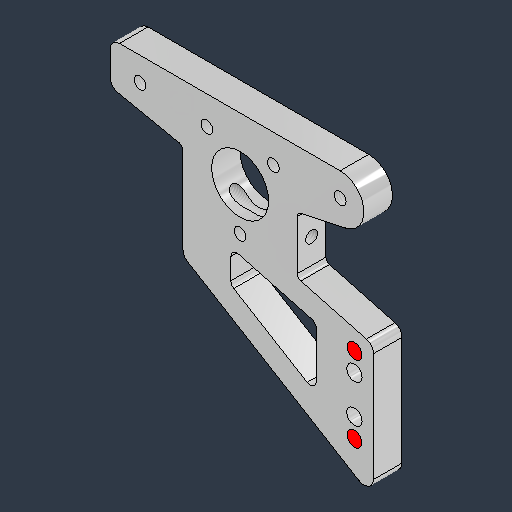
# Autodesk Inventor part: PLATE,SIDE,ELEVATOR,STAGE1
Saved by Autodesk Inventor 2024.3 (Build 283343000, 343)
## iProperties
ILogicPurgeVersion: 0.0.0.0
OnSaveVersion: 3.4.3.0
OnSaveAssembly: COREAutomationManager
Created: 2025-01-27
Part Number: PLATE,SIDE,ELEVATOR,STAGE1
Material: Aluminum 7075
Document SubType Name: Modeling
Designer: Jthib
Density: 2.81 g/cm^3
Appearance: Aluminum - Polished
Mfg Approved By: John.Thibert
Sheet Metal Rule: Default
Mass: 86.4188 g
Surface Area: 127.948 cm^2
Volume: 30.754 cm^3
ModelCat: Uncategorized
MaterialName: Aluminum 7075
CN_MASS: 0.09
Author: Jthib
Autodesk Inventor part; units mm, degrees
ref_plane "YZ Plane" through (0, 0, 0) normal (1, 0, 0) x (0, 1, 0)
ref_plane "XZ Plane" through (0, 0, 0) normal (0, 1, 0) x (-1, 0, 0)
ref_plane "XY Plane" through (0, 0, 0) normal (0, 0, 1) x (1, 0, 0)
sketch "Sketch1" plane through (0, 0, 0) normal (0, 0, 1) x (1, 0, 0)
  line L0 (33.401, 0) -> (-33.401, 0) construction
  arc A0 (33.401, 7.9375) -> (35.033, -7.7679) centre (33.401, 0) ccw construction
  arc A1 (-35.033, -7.7679) -> (-33.401, 7.9375) centre (-33.401, 0) ccw construction
  line L1 (33.401, 7.9375) -> (-33.401, 7.9375)
  line L2 (35.033, -7.7679) -> (19.1135, -11.1125)
  line L3 (19.1135, -11.1125) -> (19.1135, -30.1625)
  line L4 (19.1135, -30.1625) -> (44.5135, -36.9684)
  line L5 (44.5135, -36.9684) -> (44.5135, -81.4184)
  line L6 (44.5135, -81.4184) -> (-19.1135, -42.8625)
  line L7 (-19.1135, -42.8625) -> (-19.1135, -11.1125)
  line L8 (-19.1135, -11.1125) -> (-43.434, -6.0029)
  arc A2 (35.033, -7.7679) -> (33.401, 7.9375) centre (33.401, 0) ccw
  arc A3 (-33.401, 7.9375) -> (-35.033, -7.7679) centre (-33.401, 0) ccw
  line L9 (0, 26.6914) -> (0, -99.4367) construction
  line L10 (-33.401, 7.9375) -> (-43.434, 7.9375)
  line L11 (-43.434, 7.9375) -> (-43.434, -6.0029)
  point P0 (0, 0)
  point P1 (0, 0)
  point P2 (19.1135, -20.6375)
  dimension "d24" = 50.927
  dimension "d25" = 7.9375
  dimension "d26" = 19.05
  dimension "d27" = 19.05
  dimension "d28" = 105
  dimension "d30" = 6.35
  dimension "d31" = 44.45
  dimension "d72" = 28.575
  dimension "d110" = 31.75
  dimension "d127" = 10.033
  constraints: 22 end point, 8 point on circle, 6 tangent, 5 coincident, 4 centre point, 2 horizontal, 2 midpoint, 2 parallel, 1 equal radius, 1 perpendicular, 1 point on line, 1 vertical, 2 other
  measures "d25" radius of A2
  measures "d26" distance of L2.end L3.end
  measures "d28" angle of L3 L4
  measures "d30" distance edge to line of A0 L3
  measures "d31" distance of L4.end L5.end
  measures "d72" distance from line of L1 point (19.114, -20.638)
  measures "d110" distance of L6.end L7.end
  measures "d127" distance from line of L11 L0.end
extrude "Extrusion2" add sketch "Sketch1" along normal mid plane 9.525
sketch "Sketch2" plane through (0, 0, 4.7625) normal (0, 0, 1) x (1, 0, 0)
  arc A0 (35.033, -7.7679) -> (33.401, 7.9375) centre (33.401, 0) ccw construction
  line L0 (33.401, 0) -> (-33.401, 0) construction
  point P0 (0, 0)
  point P1 (0, 0)
  constraints: 3 coincident, 2 end point, 1 horizontal, 1 midpoint
hole "Hole1" at (33.401, 0, 4.7625) at (-33.401, 0, 4.7625) direction (0, 0, -1) diameter 3.9624 end through all thread size "10-32 UNF" class "2B" standard "ANSI Unified Screw Threads"
sketch "Sketch3" plane through (0, 0, -4.7625) normal (0, 0, -1) x (-1, 0, 0)
  line L0 (-62.103, 0) -> (61.0235, 0) construction
  line L1 (0, -99.2896) -> (0, 25.8087) construction
  line L2 (11.1125, -1.5875) -> (-11.1125, -1.5875) construction
  line L3 (0, -26.9875) -> (0, -1.5875) construction
  point P0 (0, 0)
  dimension "d43" = 22.225
  dimension "d44" = 25.4
  dimension "d45" = 1.5875
  constraints: 4 end point, 3 coincident, 1 collinear, 1 horizontal, 1 midpoint
  measures "d43" distance of L2.start L2.end
  measures "d44" distance of L3.start L3.end
  measures "d45" distance between parallel lines of L0 L2
hole "Hole2" at (0, -26.9875, -4.7625) at (11.1125, -1.5875, -4.7625) at (-11.1125, -1.5875, -4.7625) direction (0, 0, 1) diameter 3.9624 end through all thread size "10-32 UNF" class "2B" standard "ANSI Unified Screw Threads"
sketch "Sketch4" plane through (0, 0, 4.7625) normal (0, 0, 1) x (1, 0, 0)
  line L0 (0, 0) -> (0, -12.7) construction
  circle A0 centre (0, -12.7) radius 9.525
  line L1 (25.4635, -56.9863) -> (25.4635, -41.6407)
  line L2 (23.9574, -39.6779) -> (-0.5536, -33.1102)
  line L3 (-3.1115, -35.073) -> (-3.1115, -42.1335)
  line L4 (-2.1326, -43.8713) -> (22.3784, -58.7242)
  line L5 (-19.1135, -42.8625) -> (44.5135, -81.4184) construction
  line L6 (44.5135, -36.9684) -> (19.1135, -30.1625) construction
  line L7 (44.5135, -81.4184) -> (44.5135, -36.9684) construction
  arc A1 (22.3784, -58.7242) -> (25.4635, -56.9863) centre (23.4315, -56.9863) ccw
  arc A2 (25.4635, -41.6407) -> (23.9574, -39.6779) centre (23.4315, -41.6407) ccw
  arc A3 (-0.5536, -33.1102) -> (-3.1115, -35.073) centre (-1.0795, -35.073) ccw
  arc A4 (-3.1115, -42.1335) -> (-2.1326, -43.8713) centre (-1.0795, -42.1335) ccw
  point P0 (-18.2864, -30.0929)
  point P1 (20.2266, -29.9445)
  point P2 (19.1135, -30.1625)
  dimension "d54" = 19.05
  dimension "d55" = 12.7
  dimension "d56" = 19.05
  dimension "d57" = 28.575
  dimension "d58" = 7.9375
  dimension "d59" = 7.9375
  dimension "d60" = 2.032
  constraints: 10 end point, 8 point on circle, 8 tangent, 5 centre point, 3 equal radius, 2 vertical, 1 coincident, 1 parallel, 4 other
  measures "d54" diameter of A0
  measures "d55" distance of L0.start L0.end
  measures "d56" distance between parallel lines of L1 L7
  measures "d57" distance between parallel lines of L1 L3
  measures "d60" radius of A1
extrude "Extrusion3" cut sketch "Sketch4" against normal through all
sketch "Sketch6" plane through (19.1135, -30.1625, 4.7625) normal (1, 0, 0) x (0, 0, -1)
  line L0 (9.525, 19.05) -> (0, 19.05) construction
  line L1 (0, 0) -> (0, 19.05) construction
  line L2 (9.525, 0) -> (0, 0) construction
  line L3 (9.525, 19.05) -> (9.525, 0) construction
  line L4 (9.525, 0) -> (0, 19.05) construction
  point P0 (4.7625, 30.1625)
  point P1 (4.7625, 9.525)
  constraints: 2 end point, 1 midpoint
hole "Hole3" at (19.1135, -20.6375, 0) direction (-1, 0, 0) diameter 3.9624 end through all thread size "10-32 UNF" class "2B" standard "ANSI Unified Screw Threads"
sketch "Sketch8" plane through (0, 0, -4.7625) normal (0, 0, -1) x (-1, 0, 0)
  line L0 (-38.1635, -41.7309) -> (-38.1635, -48.0809) construction
  line L1 (-38.1635, -48.0809) -> (-38.1635, -60.7809) construction
  line L2 (-38.1635, -60.7809) -> (-38.1635, -67.1309) construction
  line L3 (-44.5135, -36.9684) -> (-44.5135, -81.4184) construction
  point P0 (0, 0)
  point P1 (-44.5135, -59.1934)
  point P2 (-38.1635, -54.4309)
  dimension "d85" = 12.7
  dimension "d86" = 25.4
  dimension "d88" = 4.7625
  dimension "d89" = 6.35
  constraints: 6 end point, 2 coincident, 2 collinear, 2 midpoint, 1 parallel, 1 point on line, 1 vertical
  measures "d85" distance of L0.end L1.end
  measures "d86" distance of L0.start L2.end
  measures "d88" vertical distance of point (-44.514, -59.193) point (-38.164, -54.431)
  measures "d89" distance between parallel lines of L1 L3
hole "Hole5" at (38.1635, -67.1309, -4.7625) at (38.1635, -41.7309, -4.7625) direction (0, 0, 1) diameter 5.0038 end through all clearance for "H7 - STANDARD FIT" size "5" standard "CL-DOWEL-MET"
hole "Hole6" at (38.1635, -48.0809, -4.7625) at (38.1635, -60.7809, -4.7625) direction (0, 0, 1) diameter 5.1054 end through all clearance for "Flat Head Machine Screw (82)" size "#10" standard "Ansi Unified Screw Threads"
fillet "Fillet4" radius 1.5875 3 edges at (19.1135, -30.1625, 0) (19.1135, -11.1125, 0) (-19.1135, -11.1125, 0)
fillet "Fillet5" radius 3.175 5 edges at (44.5135, -36.9684, 0) (44.5135, -81.4184, 0) (-19.1135, -42.8625, 0) (-43.434, -6.0029, 0) (-43.434, 7.9375, 0)
sketch "Sketch11" plane through (-43.434, -3.4256, -4.7625) normal (-1, 0, 0) x (0, 0, 1)
  point P0 (4.7625, 3.4256)
  point P1 (4.7625, 3.4256)
  constraints: 1 coincident
hole "Hole9" at (-43.434, 0, 0) direction (1, 0, 0) diameter 3.9624 depth 6.35 tip angle 118 thread size "10-32 UNF" class "2B" standard "ANSI Unified Screw Threads"
equation "\"d58\" = d59"
equation "\"BendRadius\" = Thickness"
equation "\"BendReliefWidth\" = Thickness"
equation "\"BendReliefDepth\" = 0.5 * Thickness"
equation "\"CornerReliefSize\" = 4 * Thickness"
equation "\"MinimumRemnant\" = 2 * Thickness"
equation "\"TransitionRadius\" = BendRadius"
equation "\"JacobiRadiusSize\" = BendRadius"
equation "\"GapSize\" = Thickness"
equation "\"Thickness\" = 6.35"
body "Solid3"
